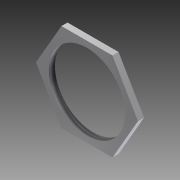
# Autodesk Inventor part: Switch Nut
Saved by Autodesk Inventor 2015 (Build 190159000, 159)
## iProperties
Created: 2015-11-02
Part Number: Switch Nut
Material: Aluminum 7075
Document SubType Name: Modeling
Designer: James
Density: 2.81 g/cm^3
Appearance: Satin - Brushed Heavy
Author: James
Autodesk Inventor part; units mm, degrees
ref_plane "YZ Plane" through (0, 0, 0) normal (1, 0, 0) x (0, 1, 0)
ref_plane "XZ Plane" through (0, 0, 0) normal (0, 1, 0) x (-1, 0, 0)
ref_plane "XY Plane" through (0, 0, 0) normal (0, 0, 1) x (1, 0, 0)
sketch "Sketch1" plane through (0, 0, 0) normal (0, 1, 0) x (-1, 0, 0)
  circle A0 centre (0, 0) radius 6.25
  line L0 (8.3716, 0) -> (4.1858, -7.25)
  line L1 (4.1858, -7.25) -> (-4.1858, -7.25)
  line L2 (-4.1858, -7.25) -> (-8.3716, 0)
  line L3 (-8.3716, 0) -> (-4.1858, 7.25)
  line L4 (-4.1858, 7.25) -> (4.1858, 7.25)
  line L5 (4.1858, 7.25) -> (8.3716, 0)
  dimension "d0" = 12.5
  dimension "d1" = 14.5
  constraints: 12 end point, 2 coincident, 1 centre point, 13 other
  measures "d0" diameter of A0
  measures "d1" distance between parallel lines of L1 L4
extrude "Extrusion1" add sketch "Sketch1" along normal blind 1
thread "Thread2" size "M14x2" class "6H" standard "ANSI Metric M Profile" full length
body "Solid1"
